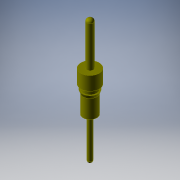
# Autodesk Inventor part: -101-G-A_pins
Saved by Autodesk Inventor 2019 (Build 230136000, 136)
## iProperties
Created: 2024-02-02
Part Number: -101-G-A_pins
Material: Generic
Catalog Web Link: www.cadenas.de
Description: TS Series Pins-TS Series - (2,54 mm) .100'' Precision Machined Terminal Strips
Vendor: SAMTEC
Document SubType Name: Modeling
Designer: psAdmin
Manufacturer: SAMTEC
Mass: 0.0088623 g
Surface Area: 0.373067 cm^2
Volume: 0.0088623 cm^3
Density: 1 g/cm^3
Appearance: PSOLRGB-255-255-0
Category: PARTsolutions
Company: SAMTEC
Title: -101-G-A_pins
Author: Cadenas PARTsolutions
Comments: TS Series - (2,54 mm) .100'' Precision Machined Terminal Strips
PSOL_IDENT_0: {$CADENAS_DATA/23d-libs/samtec/modelling/ts/parts/ts_pins.prj},186 {VTYP=3D},{NB=-101-G-A_pins},{LIN
PSOL_IDENT_1: A=-101-G-A_pins},{NN=TS Series Pins},{DATE=18.08.2016 05:41:39},{GEOMDATE=18.08.2016 05:41:00},{VERS
PSOL_IDENT_2: ION=},{LINEID=10},{WBVAR=POS,PLOPT,LS},{WBNUMERIC=}  {NB=-101-G-A_pins},{LINA=-101-G-A_pins},{KT=DUM
PSOL_IDENT_3: MY},{PN=-101-G-A},{SERIES=TS},{ROW=},{POS=01},{POSN=1},{POSALG=  '01','-01'},{POSPN=01},{PLOPTALG= '
PSOL_IDENT_4: G','-G = 20micro\" Selective Gold.'    },{PLOPT=G},{LSALG= 'AA','-AA','A','-A','A-1','-A-1','A-2','-
PSOL_IDENT_5: A-2','B','-B','B-2','-B-2','C','-C','C-1','-C-1','C-2','-C-2','D-1-1','-D-1-1','D-1-2','-D-1-2','E','
PSOL_IDENT_6: -E','G-1','-G-1','J','-J','K','-K','L-1','-L-1','L-2','-L-2','L-3','-L-3','N','-N','Q-3','-Q-3' },{L
PSOL_IDENT_7: S=A},{FIG=2},{B=0.10000},{C=0.143},{D=0.018},{D2=0.025},{E=0.156},{F=0.166},{G=0.008},{H=0.070},{I=0
PSOL_IDENT_8: .052},{J=0.052},{PL=0.477},{SQ=0.000},{W=0.10000},{X=0}
NB: -101-G-A_pins
NN: TS Series Pins
NT: TS Series - (2,54 mm) .100'' Precision Machined Terminal Strips
NBSYN: $PN._pins
LINA: -101-G-A_pins
CATALOG: Samtec
PN: -101-G-A
SERIES: TS
POS: -01
PLOPT: -G = 20micro" Selective Gold.
LS: -A
FIG: 2
B: 0.1
C: 0.143
D: 0.018
D2: 0.025
E: 0.156
F: 0.166
G: 0.008
H: 0.07
I: 0.052
J: 0.052
PL: 0.477
SQ: 0
W: 0.1
X: 0
SUPPLIER: SAMTEC
ARTICLENO: -101-G-A_pins
BOMINFO: -101-G-A_pins
CREATOR: CADENAS GmbH
Autodesk Inventor part; units mm, degrees
sketch "Sketch_1" plane through (0, 0, 0) normal (0, 0, 1) x (1, 0, 0)
  line L0 (0, -2.717) -> (0, 1.3208)
  line L1 (0, 1.3208) -> (0.889, 1.3208)
  line L2 (0.889, 1.3208) -> (0.889, 0)
  line L3 (0.889, 0) -> (0.6604, 0)
  line L4 (0.6604, 0) -> (0.6604, -0.4572)
  line L5 (0.6604, -0.4572) -> (0.7747, -0.4572)
  line L6 (0.7747, -0.4572) -> (0.6604, -0.7712)
  line L7 (0.6604, -0.7712) -> (0.6604, -2.54)
  line L8 (0.6604, -2.54) -> (0, -2.717)
  line L9 (0, -2.717) -> (0, 1.3208)
  constraints: 20 end point
revolve "Revolution1" add sketch "Sketch_1" angle 360 about axis through (0, -2.717, 0) along (0, -1, 0)
sketch "Sketch_3" plane through (0, 0, 0) normal (0, 0, 1) x (1, 0, 0)
  line L0 (0, 1.3208) -> (0, 5.5372)
  line L1 (0, 5.5372) -> (0.0508, 5.5372)
  arc A0 (0.3175, 5.2705) -> (0.0508, 5.5372) centre (0.0508, 5.2705) ccw
  line L2 (0.3175, 5.2705) -> (0.3175, 1.3208)
  line L3 (0.3175, 1.3208) -> (0, 1.3208)
  line L4 (0, 1.3208) -> (0, 5.5372)
  constraints: 10 end point, 2 point on circle, 1 centre point
revolve "Revolution2" add sketch "Sketch_3" angle 360 about axis through (0, 1.3208, 0) along (0, -1, 0)
sketch "Sketch_14" plane through (0, 0, 0) normal (0, 0, 1) x (1, 0, 0)
  line L0 (0, -6.5786) -> (0, -1.6256)
  line L1 (0, -1.6256) -> (0.2286, -1.6256)
  line L2 (0.2286, -1.6256) -> (0.2286, -6.4008)
  arc A0 (0.0508, -6.5786) -> (0.2286, -6.4008) centre (0.0508, -6.4008) ccw
  line L3 (0.0508, -6.5786) -> (0, -6.5786)
  line L4 (0, -6.5786) -> (0, -1.6256)
  constraints: 10 end point, 2 point on circle, 1 centre point
revolve "Revolution3" add sketch "Sketch_14" angle 360 about axis through (0, -6.5786, 0) along (0, -1, 0)
ref_plane "pins_XY" through (0, 0, 0) normal (0, 1, 0) x (1, 0, 0)
ref_plane "pins_YZ" through (0, 0, 0) normal (1, 0, 0) x (0, 0, -1)
ref_plane "pins_ZX" through (0, 0, 0) normal (0, 0, -1) x (0, 1, 0)
body "Solid1"
